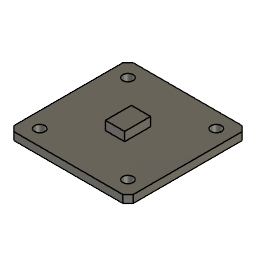
MT6701 (Autodesk Fusion 360 design; units mm, degrees)
Autodesk Fusion 360 part; units mm, degrees
sketch "Sketch1" plane through (0, 0, 0) normal (0, 0, 1) x (1, 0, 0)
  line L0 (11.5, 11.5) -> (-11.5, 11.5)
  line L1 (-11.5, 11.5) -> (-11.5, -11.5)
  line L2 (-11.5, -11.5) -> (11.5, -11.5)
  line L3 (11.5, -11.5) -> (11.5, 11.5)
  line L4 (11.5, 11.5) -> (-11.5, -11.5) construction
  line L5 (-11.5, 11.5) -> (11.5, -11.5) construction
  dimension "d1" = 23
  dimension "d2" = 23
  constraint horizontal L0
  constraint perpendicular L0 L1
  constraint parallel L0 L2
  constraint parallel L1 L3
  constraint coincident L4 origin
  constraint coincident L5 origin
  measures "d1" distance of L1.end L2.end
  measures "d2" distance of L0.end L1.end
extrude "Extrude1" add sketch "Sketch1" along normal blind 1.5
chamfer "Chamfer1" distance 1 angle 45 4 edges at (-11.5, -11.5, 0.75) (11.5, -11.5, 0.75) (11.5, 11.5, 0.75) (-11.5, 11.5, 0.75)
sketch "Sketch2" plane through (0, 0, 1.5) normal (0, 0, 1) x (-1, 0, 0)
  line L0 (10.5, -11.5) -> (11.5, -10.5)
  line L1 (11.5, -10.5) -> (11.5, 10.5)
  line L2 (11.5, 10.5) -> (10.5, 11.5)
  line L3 (10.5, 11.5) -> (-10.5, 11.5)
  line L4 (-10.5, 11.5) -> (-11.5, 10.5)
  line L5 (-11.5, 10.5) -> (-11.5, -10.5)
  line L6 (-11.5, -10.5) -> (-10.5, -11.5)
  line L7 (-10.5, -11.5) -> (10.5, -11.5)
  line L8 (-1.85, 2.5) -> (1.85, 2.5)
  line L9 (1.85, 2.5) -> (1.85, -2.5)
  line L10 (1.85, -2.5) -> (-1.85, -2.5)
  line L11 (-1.85, -2.5) -> (-1.85, 2.5)
  line L12 (-1.85, 2.5) -> (1.85, -2.5) construction
  line L13 (1.85, 2.5) -> (-1.85, -2.5) construction
  dimension "d6" = 3.7
  dimension "d7" = 5
  constraint horizontal L8
  constraint perpendicular L8 L9
  constraint parallel L8 L10
  constraint parallel L9 L11
  constraint coincident L12 origin
  constraint coincident L13 origin
  measures "d6" distance of L9.end L10.end
  measures "d7" distance of L8.end L9.end
extrude "Extrude2" add sketch "Sketch2" along normal blind 1.7 contours L8 L9 L10 L11
sketch "Sketch3" plane through (0, 0, 1.5) normal (0, 0, 1) x (-1, 0, 0)
  line L0 (-1.85, -2.5) -> (-1.85, 2.5)
  line L1 (-1.85, 2.5) -> (1.85, 2.5)
  line L2 (1.85, 2.5) -> (1.85, -2.5)
  line L3 (1.85, -2.5) -> (-1.85, -2.5)
  line L4 (10.5, -11.5) -> (11.5, -10.5)
  line L5 (11.5, -10.5) -> (11.5, 10.5)
  line L6 (11.5, 10.5) -> (10.5, 11.5)
  line L7 (10.5, 11.5) -> (-10.5, 11.5)
  line L8 (-10.5, 11.5) -> (-11.5, 10.5)
  line L9 (-11.5, 10.5) -> (-11.5, -10.5)
  line L10 (-11.5, -10.5) -> (-10.5, -11.5)
  line L11 (-10.5, -11.5) -> (10.5, -11.5)
  line L12 (-8.5, -8.5) -> (8.5, -8.5) construction
  line L13 (8.5, -8.5) -> (8.5, 8.5) construction
  line L14 (8.5, 8.5) -> (-8.5, 8.5) construction
  line L15 (-8.5, 8.5) -> (-8.5, -8.5) construction
  line L16 (-8.5, -8.5) -> (8.5, 8.5) construction
  line L17 (8.5, -8.5) -> (-8.5, 8.5) construction
  circle A0 centre (8.5, -8.5) radius 1
  circle A1 centre (-8.5, -8.5) radius 1
  circle A2 centre (-8.5, 8.5) radius 1
  circle A3 centre (8.5, 8.5) radius 1
  dimension "d10" = 2
  dimension "d11" = 17
  constraint horizontal L12
  constraint perpendicular L12 L13
  constraint parallel L12 L14
  constraint parallel L13 L15
  constraint coincident L16 origin
  constraint coincident L17 origin
  constraint equal L12 L15
  constraint coincident L12.end L13.start
  constraint coincident L12.start L15.end
  constraint coincident L14.end L15.start
  constraint coincident L13.end L14.start
  constraint equal A2 A3
  constraint equal A1 A2
  constraint equal A0 A1
  measures "d10" diameter of A0
  measures "d11" distance of L12.start L12.end
extrude "Extrude3" cut sketch "Sketch3" against normal up to surface (1.5 mm away) contours A0 | A1 | A2 | A3
equation "d8 = 3.2 mm - 1.5 mm"
